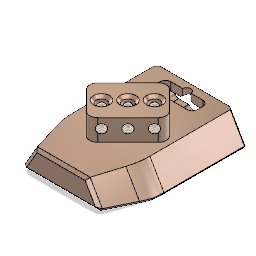
Specimen Puck - Regular v11 (Autodesk Fusion 360 archive; units mm, degrees)
design "specimen puck regular"
Autodesk Fusion 360 part; units mm, degrees
sketch "Sketch1" plane through (0, 0, 0) normal (0, 0, 1) x (1, 0, 0)
  line L0 (10, 0) -> (-10, 0)
  line L1 (-10, 0) -> (-7.1132, 5)
  line L2 (-7.1132, 5) -> (7.1132, 5)
  line L3 (7.1132, 5) -> (10, 0)
  line L4 (0, 2.5) -> (0, 20)
  line L5 (-8.5566, 2.5) -> (8.5566, 2.5) construction
  line L6 (4, 3.5) -> (4, 1.5)
  line L7 (4, 3.5) -> (-4, 3.5)
  line L8 (-4, 3.5) -> (-4, 1.5)
  line L9 (-4, 1.5) -> (4, 1.5)
  line L10 (7.1132, 5) -> (0, 17.3205)
  dimension "d1" = 20
  dimension "d2" = 5
  dimension "d3" = 60
  dimension "d5" = 8
  dimension "d7" = 2
  constraint horizontal L0
  constraint parallel L0 L2
  constraint coincident origin L0
  constraint symmetric L1 L3 L4
  constraint midpoint L1 L5.start
  constraint midpoint L3 L5.end
  constraint perpendicular L5 L6
  constraint parallel L5 L7
  constraint perpendicular L5 L8
  constraint perpendicular L8 L9
  constraint symmetric L4 L6 L8
  constraint coincident L6.start L7.start
  constraint coincident L6.end L9.end
  constraint symmetric L5 L7 L9
  constraint coincident L4 L10.end
  constraint collinear L3 L10
  measures "d1" distance of L0.start L0.end
  measures "d2" distance of L0 L2
  measures "d3" angle of L1 L3
  measures "d5" distance of L6 L8
  measures "d7" distance of L7 L9
extrude "Extrude1" add sketch "Sketch1" along normal blind 25 contours L0 L1 L2 L3 | L6 L7 L8 L9
sketch "Sketch2" plane through (0, 0, 0) normal (0, 1, 0) x (1, 0, 0)
  line L0 (-4, -4.5) -> (4, -4.5)
  line L1 (4, -4.5) -> (4, -1.5)
  line L2 (4, -1.5) -> (-4, -1.5)
  line L3 (-4, -1.5) -> (-4, -4.5)
  line L4 (10, 0) -> (-10, 0)
  line L5 (0, -1.75) -> (0, -22.5) construction
  line L6 (-7.1132, -25.2701) -> (7.1132, -11.0436)
  line L7 (7.1132, 0) -> (7.1132, -25)
  line L8 (-7.1132, 0) -> (-7.1132, -25)
  line L9 (-7.1132, -13.9564) -> (7.1132, 0.2701)
  line L10 (-2.4749, -14.9749) -> (2.4749, -10.0251)
  line L11 (-6.7175, -13.5607) -> (-1.0607, -19.2175)
  line L12 (6.7175, -11.4393) -> (1.0607, -5.7825)
  point P0 (-4, 0)
  point P1 (4, 0)
  point P2 (0, -1.5)
  point P3 (0, -12.5)
  dimension "d10" = 3
  dimension "d11" = 1.5
  dimension "d27" = 12.5
  dimension "d82" = 45
  dimension "d85" = 7
  dimension "d95" = 2
  dimension "d96" = 2
  dimension "d97" = 8
  constraint horizontal L0
  constraint vertical L1
  constraint horizontal L2
  constraint vertical L3
  constraint coincident L1 P1
  constraint coincident L3 P0
  constraint midpoint L2 P2
  constraint coincident L5 P3
  constraint coincident L6.start L8
  constraint coincident L6.end L7
  constraint coincident L7 L9.end
  constraint parallel L6 L9
  constraint parallel L6 L10
  constraint midpoint P3 L10
  constraint coincident L8 L9.start
  constraint coincident L9 L11.start
  constraint coincident L6 L11.end
  constraint perpendicular L6 L11
  constraint coincident L6 L12.start
  constraint coincident L9 L12.end
  constraint perpendicular L9 L12
  measures "d10" distance of L0 L2
  measures "d11" distance of L2 L4
  measures "d27" distance of origin P3
  measures "d82" angle of L4 L9
  measures "d85" distance of L10.start L10.end
  measures "d95" distance of L10.start L11
  measures "d96" distance of L10.end L12
  measures "d97" distance of L6 L9
sketch "Sketch3" plane through (0, 5, 0) normal (0, 1, 0) x (-1, 0, 0)
  line L0 (-7.1132, 0) -> (7.1132, 0)
  line L1 (7.1132, 0) -> (7.1132, 25)
  line L2 (7.1132, 25) -> (-7.1132, 25)
  line L3 (-7.1132, 25) -> (-7.1132, 0)
  point P0 (0, 12.5)
hole "Hole1" at (0, 2.5, 0) direction (0, 0, 1) diameter 3 depth 12 tip angle 118
hole "Hole2" at (0, 0, 1.5) direction (0, 1, 0) diameter 1.5 end through all
extrude "Extrude2" cut sketch "Sketch1" along normal blind 3.5 contours L6 L7 L8 L9
extrude "Extrude3" cut sketch "Sketch2" along normal through all contours L0 L1 L2 L3 L9 | L0 L1 L9
ref_plane "WorkPlane1" through (0, 2.5, 17.5) normal (0, 0, 1) x (1, 0, 0)
split_face "SplitFace1" 3 faces at (8.0755, 3.3333, 8.3333) (-1.3333, 0, 18.1667) (-9.0377, 1.6667, 8.3333) by plane through (0, 2.5, 17.5) normal (0, 0, 1)
draft "Draft1" angle 15 neutral plane through (0, 2.5, 17.5) pull (0, 0, 1) 2 faces at (8.0755, 3.3333, 20) (-9.0377, 1.6667, 20)
draft "Draft2" angle 5 neutral plane through (0, 2.5, 17.5) pull (0, 0, 1) 1 faces at (-2.5598, 0, 20)
extrude "Extrude9" add sketch "Sketch2" along normal blind 4 from surface at 5 contours L6 L9 L11 L12
hole "Hole10" at (2.4749, 0, 10.0251) at (0, 0, 12.5) at (-2.4749, 0, 14.9749) direction (0, 1, 0) diameter 2 end through all
sketch "Sketch9" plane through (3.4216, 0, 3.4216) normal (-0.707107, 0, -0.707107) x (-0.707107, 0, 0.707107)
  line L0 (3.3388, 5) -> (14.3388, 5)
  line L1 (14.3388, 5) -> (14.3388, 9)
  line L2 (14.3388, 9) -> (3.3388, 9)
  line L3 (3.3388, 9) -> (3.3388, 5)
  line L4 (4.3388, 9) -> (6.3388, 9)
  line L5 (7.8388, 9) -> (9.8388, 9)
  line L6 (11.3388, 9) -> (13.3388, 9)
  line L7 (5.3388, 9) -> (5.3388, 7.2)
  line L8 (8.8388, 9) -> (8.8388, 7.2)
  line L9 (12.3388, 9) -> (12.3388, 7.2)
  dimension "d98" = 2.2
  constraint midpoint L4 L7.start
  constraint perpendicular L2 L7
  constraint midpoint L2 L8.start
  constraint perpendicular L2 L8
  constraint midpoint L6 L9.start
  constraint perpendicular L2 L9
  constraint horizontal L7.end L8.end
  constraint horizontal L8.end L9.end
  measures "d98" distance of L0 L9.end
hole "Hole11" at (-0.3536, 7.2, 7.1967) at (-2.8284, 7.2, 9.6716) at (-5.3033, 7.2, 12.1464) direction (0.707107, 0, 0.707107) diameter 1.623 end through all
thread "Thread4" "ISO Metric profile 2.0 M2x0.4 6H" major diameter 2.074 minor diameter 1.623 pitch 0.4 angle 60 resizes the face on face at (1.4964, 7.8204, 8.3069) on face at (5.072, 7.1985, 11.4747) on face at (-0.9785, 7.8204, 10.7818) on face at (2.5972, 7.1985, 13.9495) on face at (-3.4533, 7.8204, 13.2567) on face at (0.1223, 7.1985, 16.4244)
fillet "Fillet5" radius 1.5 4 edges at (-6.7175, 7, 13.5607) (-1.0607, 7, 19.2175) (1.0607, 7, 5.7825) (6.7175, 7, 11.4393)
fillet "Fillet2" radius 15 2 edges at (8.5566, 2.5, 17.5) (-8.5566, 2.5, 17.5)
chamfer "Chamfer1" distance 0.5 angle 45 14 edges at (0, 5, 25) (-6.0467, 2.8281, 25) (0, 0.6562, 25) (6.0467, 2.8281, 25) (8.3071, 0.4115, 22.2037) (9.6168, 0.084, 18.4599) (9.9623, 0, 16.5148) (10, 0, 7.7626) (8.5566, 2.5, 0) (-9.6168, 0.084, 18.4599) (-8.3071, 0.4115, 22.2037) (-10, 0, 7.7626) (-9.9623, 0, 16.5148) (-8.5566, 2.5, 0)
fillet "Fillet1" radius 1 10 edges at (-4, 2.5, 4.5) (-4, 4.25, 1.5) (-4, 0.75, 1.5) (4, 4.25, 1.5) (4, 0.75, 1.5) (4, 2.5, 4.5) (4, 1.5, 0.75) (4, 3.5, 0.75) (-4, 3.5, 0.75) (-4, 1.5, 0.75)
chamfer "Chamfer6" distance 0.5 angle 45 6 edges at (2.1133, 9, 10.9575) (-0.3616, 9, 13.4323) (-2.8365, 9, 15.9072) (-2.1133, 0, 15.9072) (0.3616, 0, 13.4323) (2.8365, 0, 10.9575)
